LED Design-Body (Autodesk Fusion 360 design; units mm, degrees)
Autodesk Fusion 360 part; units mm, degrees
note: some values were not read from the file. Chosen so that the rebuilt part matches the saved one: which face or edge a step refers to.
sketch "Sketch1" plane through (0, 0, 0) normal (0, 1, 0) x (1, 0, 0)
  line L0 (47, 36) -> (-47, 36)
  line L1 (-47, 36) -> (-47, -36)
  line L2 (-47, -36) -> (47, -36)
  line L3 (47, -36) -> (47, 36)
  line L4 (47, 36) -> (-47, -36) construction
  line L5 (-47, 36) -> (47, -36) construction
  dimension "d1" = 72
  dimension "d2" = 94
  measures "d1" distance of L0.start L1.end
  measures "d2" distance of L0.start L0.end
extrude "Extrude1" add sketch "Sketch1" along normal blind 60
sketch "Sketch2" plane through (0, 60, 0) normal (0, 1, 0) x (-1, 0, 0)
  line L0 (-47, 36) -> (-47, -36)
  line L1 (-47, -36) -> (47, -36)
  line L2 (47, -36) -> (47, 36)
  line L3 (47, 36) -> (-47, 36)
  line L4 (42, -31) -> (11, -31)
  line L5 (11, -31) -> (11, 31)
  line L6 (11, 31) -> (42, 31)
  line L7 (42, 31) -> (42, -31)
  line L8 (8, -31) -> (-42, -31)
  line L9 (-42, -31) -> (-42, 31)
  line L10 (-42, 31) -> (8, 31)
  line L11 (8, 31) -> (8, -31)
  dimension "d5" = 31
  dimension "d6" = 62
  dimension "d7" = 5
  dimension "d8" = 5
  dimension "d9" = 50
  dimension "d10" = 62
  dimension "d11" = 5
  dimension "d12" = 5
  measures "d5" distance of L4.start L4.end
  measures "d6" distance of L4.start L6.end
  measures "d7" distance of L2 L7
  measures "d8" distance of L1 L4
  measures "d9" distance of L8.start L8.end
  measures "d10" distance of L8.end L9.end
  measures "d11" distance of L1 L8
  measures "d12" distance of L0 L9
extrude "Extrude2" cut sketch "Sketch2" against normal blind 55 contours L4 L5 L6 L7 | L8 L9 L10 L11
sketch "Sketch3" plane through (-8, 0, 0) normal (1, 0, 0) x (0, 0, -1)
  line L0 (31, 60) -> (-31, 60)
  line L1 (-31, 60) -> (-31, 5)
  line L2 (-31, 5) -> (31, 5)
  line L3 (31, 5) -> (31, 60)
  line L4 (31, 40.2906) -> (31, 25)
  line L5 (17.9771, 25) -> (14.0458, 32.6453)
  line L6 (14.0458, 32.6453) -> (17.9771, 39.9065)
  line L7 (17.9771, 39.9065) -> (31, 40.2906)
  line L8 (31, 25) -> (17.9771, 25)
  line L9 (31, 25) -> (31, 40.2906)
extrude "Extrude3" cut sketch "Sketch3" against normal blind 20 contours L3 L4 L5 L6 L7 L8 L9
sketch "Sketch4" plane through (0, 5, 0) normal (0, 1, 0) x (-1, 0, 0)
  line L0 (8, 31) -> (-42, 31)
  line L1 (-42, 31) -> (-42, -31)
  line L2 (-42, -31) -> (8, -31)
  line L3 (8, -31) -> (8, 31)
  point P0 (4.75, -26.7449)
  point P1 (-38.75, -26.5)
  point P2 (-38.7287, 17)
  point P3 (4.7713, 16.7551)
  point P4 (4.75, -26.7449)
  point P5 (4.7713, 16.7551)
  point P6 (-38.7287, 17)
  dimension "d20" = 43.5
  dimension "d21" = 43.5
  dimension "d22" = 43.5
  dimension "d23" = 43.5
  dimension "d24" = 3.25
  dimension "d25" = 4.5
  measures "d20" distance of P4 P3
  measures "d21" distance of P4 P1
  measures "d22" distance of P1 P2
  measures "d23" distance of P6 P5
  measures "d24" distance of L3 P4
  measures "d25" distance of L2 P1
sketch "Sketch5" plane through (17, 5, 0) normal (0, 1, 0) x (-1, 0, 0)
fillet "Fillet1" radius 3 3 edges at (-9.5, 39.9065, -17.9771) (-9.5, 25, -17.9771) (-9.5, 32.6453, -14.0458)
cylinder "CylinderPrimitive5" add diameter 2.2 height 15 placed x (1, 0, 0) y (0, 0, -1) z (0, 1, 0) at (-4.75, 5, -26.7449)
cylinder "CylinderPrimitive6" add diameter 2.2 height 15 placed x (1, 0, 0) y (0, 0, -1) z (0, 1, 0) at (38.7576, 5, -26.4506)
cylinder "CylinderPrimitive7" add diameter 2.2 height 15 placed x (1, 0, 0) y (0, 0, -1) z (0, 1, 0) at (-4.7713, 5, 16.7551)
cylinder "CylinderPrimitive8" add diameter 2.2 height 15 placed x (1, 0, 0) y (0, 0, -1) z (0, 1, 0) at (38.7287, 5, 17)
fillet "Fillet8" radius 2 1 edges at (-5.7756, 5, -27.1427)
fillet "Fillet9" radius 2 1 edges at (37.7321, 5, -26.8483)
fillet "Fillet10" radius 2 1 edges at (37.7031, 5, 16.6022)
fillet "Fillet11" radius 2 1 edges at (-5.7969, 5, 16.3573)
fillet "Fillet12" radius 1 1 edges at (-5.7969, 20, 17.1529)
fillet "Fillet13" radius 1 3 edges at (-5.7756, 20, -26.3471) (37.7321, 20, -26.0528) (37.7031, 20, 17.3978)
fillet "Fillet14" radius 3 1 edges at (47, 30, -36)
fillet "Fillet15" radius 3 3 edges at (-47, 30, -36) (-47, 30, 36) (47, 30, 36)
sketch "Sketch14" plane through (0, 0, 31) normal (0, 0, -1) x (-1, 0, 0)
  line L0 (8, 60) -> (-42, 60)
  line L1 (-42, 60) -> (-42, 5)
  line L2 (-42, 5) -> (8, 5)
  line L3 (8, 5) -> (8, 60)
  point P0 (8, 60)
  point P1 (8, 49.3783)
  point P2 (8, 49.3783)
  point P3 (8, 49.3783)
  point P4 (10, 0)
extrude "Extrude5" cut 1 faces at (-8, 32.4777, 15.8524) along direction (-1, 0, 0) blind 5
sketch "Sketch15" plane through (0, 5, 0) normal (0, 1, 0) x (-1, 0, 0)
  circle A0 centre (4.7713, 16.7551) radius 3.1
  circle A1 centre (-38.7576, -26.4506) radius 3.1
  circle A2 centre (4.75, -26.7449) radius 3.1
  circle A3 centre (-38.7287, 17) radius 3.1
  line L0 (-42, -31) -> (42, -31)
  line L1 (42, -31) -> (42, 31)
  line L2 (42, 31) -> (-42, 31)
  line L3 (-42, 31) -> (-42, -31)
  line L4 (11, -31) -> (8, -31)
  line L5 (8, -31) -> (8, 31)
  line L6 (8, 31) -> (11, 31)
  line L7 (11, 31) -> (11, -31)
  point P0 (8, 31)
  dimension "d62" = 3
  measures "d62" distance of L5 L7
extrude "Extrude6" add sketch "Sketch15" along normal blind 45 contours L0 L2 L4 L5 L6 L7
sketch "Sketch16" plane through (0, 60, 0) normal (0, 1, 0) x (-1, 0, 0)
  line L0 (42, -31) -> (-42, -31)
  line L1 (-42, -31) -> (-42, 31)
  line L2 (-42, 31) -> (42, 31)
  line L3 (42, 31) -> (42, -31)
  arc A0 (-44, 36) -> (-47, 33) centre (-44, 33) ccw
  line L4 (-47, 33) -> (-47, -33)
  arc A1 (-47, -33) -> (-44, -36) centre (-44, -33) ccw
  line L5 (-44, -36) -> (44, -36)
  arc A2 (44, -36) -> (47, -33) centre (44, -33) ccw
  line L6 (47, -33) -> (47, 33)
  arc A3 (47, 33) -> (44, 36) centre (44, 33) ccw
  line L7 (44, 36) -> (-44, 36)
  line L8 (11, -31) -> (8, -31)
  line L9 (8, -31) -> (8, 31)
  line L10 (8, 31) -> (11, 31)
  line L11 (11, 31) -> (11, -31)
  point P0 (11, -31)
  point P1 (11, -31)
  point P2 (8, -31)
  point P3 (8, -31)
  point P4 (8, 31)
  point P5 (8, 31)
  point P6 (11, 31)
  point P7 (11, 31)
extrude "Extrude8" cut sketch "Sketch16" against normal blind 11 contours L0 L2 L8 L9 L10 L11
sketch "Sketch17" plane through (0, 0, 36) normal (0, 0, 1) x (1, 0, 0)
  line L0 (44, 0) -> (44, 60)
  line L1 (44, 60) -> (-44, 60)
  line L2 (-44, 60) -> (-44, 0)
  line L3 (-44, 0) -> (44, 0)
  line L4 (-44, 60) -> (44, 60)
  line L5 (-12.4, 49.2) -> (12.4, 49.2)
  line L6 (12.4, 49.2) -> (12.4, 51.3)
  line L7 (12.4, 51.3) -> (-12.4, 51.3)
  line L8 (-12.4, 51.3) -> (-12.4, 49.2)
  point P0 (-12.4, 49.2)
  point P1 (-12.4, 51.3)
  point P2 (12.4, 51.3)
  point P3 (12.4, 49.2)
  dimension "d63" = 8.7
  dimension "d64" = 31.6
  dimension "d65" = 2.1
  dimension "d66" = 31.6
  dimension "d67" = 31.6
  dimension "d68" = 31.6
  dimension "d69" = 8.7
  dimension "d70" = 2.1
  measures "d63" distance of P1 L4
  measures "d64" distance of L2 P1
  measures "d65" distance of P0 P1
  measures "d66" distance of L2 P0
  measures "d67" distance of L0 P2
  measures "d68" distance of L0 P3
  measures "d69" distance of P2 L4
  measures "d70" distance of P2 P3
extrude "Extrude7" cut sketch "Sketch17" along normal blind 66 from surface at -69 contours L5 L6 L7 L8
extrude "Extrude9" cut 1 faces at (-10, 49, 10.3333) along direction (0, -1, 0) blind 0.2
extrude "Extrude10" add 1 faces at (-10, 48.8, 10.3333) along direction (0, 1, 0) blind 0.3
extrude "Extrude11" cut 1 faces at (-10, 49.1, 10.3333) along direction (0, -1, 0) blind 0.5
extrude "Extrude12" cut 1 faces at (-10, 48.6, 10.3333) along direction (0, -1, 0) blind 0.5
extrude "Extrude13" cut 1 faces at (-10, 48.1, 10.3333) along direction (0, -1, 0) blind 0.5
extrude "Extrude14" cut 1 faces at (-10, 47.6, 10.3333) along direction (0, -1, 0) blind 2
extrude "Extrude15" cut 1 faces at (-10, 45.6, 10.3333) along direction (0, -1, 0) blind 3
sketch "Sketch18" plane through (-11, 0, 0) normal (-1, 0, 0) x (0, 0, 1)
  line L0 (31, 42.6) -> (-31, 42.6)
  line L1 (-31, 42.6) -> (-31, 5)
  line L2 (-31, 5) -> (31, 5)
  line L3 (31, 5) -> (31, 42.6)
  point P0 (-31, 28.4172)
  point P1 (-31, 21.9688)
sketch "Sketch19" plane through (-8, 0, 0) normal (1, 0, 0) x (0, 0, -1)
  line L0 (31, 42.6) -> (-31, 42.6)
  line L1 (-31, 42.6) -> (-31, 5)
  line L2 (-31, 5) -> (31, 5)
  line L3 (31, 5) -> (31, 42.6)
  line L4 (-31, 30.9802) -> (-18.487, 30.9802)
  line L5 (-18.487, 30.9802) -> (-18.487, 19.9802)
  line L6 (-18.487, 19.9802) -> (-31, 19.9802)
  line L7 (-31, 19.9802) -> (-31, 30.9802)
  dimension "d90" = 11
  measures "d90" distance of L4.start L6.end
extrude "Extrude16" cut sketch "Sketch19" against normal blind 5 contours L1 L4 L5 L6 L7
chamfer "Chamfer1" distance 5.5 angle 45 1 edges at (-9.5, 30.9802, 18.487)
chamfer "Chamfer2" distance 5.5 angle 45 1 edges at (-9.5, 19.9802, 18.487)
fillet "Fillet16" radius 2 4 edges at (-9.5, 25.4791, 18.487) (-9.5, 25.4802, 18.487) (-9.5, 19.9802, 23.9859) (-9.5, 30.9802, 23.987)
sketch "Sketch20" plane through (0, 5, 0) normal (0, 1, 0) x (-1, 0, 0)
  line L0 (11, 31) -> (11, -31)
  line L1 (11, -31) -> (42, -31)
  line L2 (42, -31) -> (42, 31)
  line L3 (42, 31) -> (11, 31)
  line L4 (20, -21.5) -> (32.4559, -21.5)
  line L5 (32.4559, -21.5) -> (32.4559, -25.8568)
  line L6 (32.4559, -25.8568) -> (20, -25.8568)
  line L7 (20, -25.8568) -> (20, -21.5)
  point P0 (20, -21.5)
  point P1 (32.4559, -21.5)
  dimension "d96" = 52.5
  dimension "d97" = 52.5
  measures "d96" distance of L3 P0
  measures "d97" distance of L3 P1
extrude "Extrude17" add sketch "Sketch20" along normal blind 21 contours L4 L5 L6 L7
sketch "Sketch21" plane through (0, 0, -21.5) normal (0, 0, 1) x (1, 0, 0)
  line L0 (-32.4559, 5) -> (-20, 5)
  line L1 (-20, 5) -> (-20, 26)
  line L2 (-20, 26) -> (-32.4559, 26)
  line L3 (-32.4559, 26) -> (-32.4559, 5)
  line L4 (-32.4559, 26) -> (-20, 26)
  line L5 (-20, 26) -> (-20, 22.2)
  line L6 (-20, 22.2) -> (-32.4559, 22.2)
  line L7 (-32.4559, 22.2) -> (-32.4559, 26)
  point P0 (-32.4559, 26)
  point P1 (-20, 26)
  dimension "d100" = 3.8
  measures "d100" distance of P0 L6.end
extrude "Extrude18" add sketch "Sketch21" along normal blind 2 contours L1 L2 L3 L4 L5 L6 L7
fillet "Fillet17" radius 2 1 edges at (-26.228, 26, -25.8568)
chamfer "Chamfer3" distance 1 angle 45 1 edges at (-26.228, 22.2, -19.5)
other "CylinderPrimitive1"
other "CylinderPrimitive2"
other "CylinderPrimitive3"
other "CylinderPrimitive4"
fillet "Fillet2" [suppressed]
fillet "Fillet3" [suppressed]
fillet "Fillet4" [suppressed]
fillet "Fillet5" [suppressed]
fillet "Fillet6" [suppressed]
fillet "Fillet7" [suppressed]
sketch "Sketch9" plane through (0, 60, 0) normal (0, 1, 0) x (-1, 0, 0)
  line L0 (-42, -31) -> (-42, 31)
  line L1 (-42, 31) -> (8, 31)
  line L2 (8, 31) -> (8, -31)
  line L3 (8, -31) -> (-42, -31)
  line L4 (11, -31) -> (11, 31)
  line L5 (11, 31) -> (42, 31)
  line L6 (42, 31) -> (42, -31)
  line L7 (42, -31) -> (11, -31)
  line L8 (-47, 36) -> (-47, -36)
  line L9 (-47, -36) -> (47, -36)
  line L10 (47, -36) -> (47, 36)
  line L11 (47, 36) -> (-47, 36)
  line L12 (11, -31) -> (11, 31)
  line L13 (11, 31) -> (11, -31)
  line L14 (8, -31) -> (8, 31)
  line L15 (11, 31) -> (11, -31)
  line L16 (8, -31) -> (11, -31)
  line L17 (8, 31) -> (11, 31)
  line L18 (11, -31) -> (11, 31)
  line L19 (8, 31) -> (8, -31)
  point P0 (11, 31)
  point P1 (11, -31)
  point P2 (8, -31)
  point P3 (8, 31)
  point P4 (8, 31)
extrude "Extrude4" [suppressed]
sketch "Sketch10" plane through (0, 0, 0) normal (1, 0, 0) x (0, 0, -1)
  point P0 (17.8766, -6.9109)
  point P1 (-67.1615, 47.9414)
component "Component" placed x (1, 0, 0) y (0, 1, 0) z (0, 0, 1) at (0, 0, 0)
